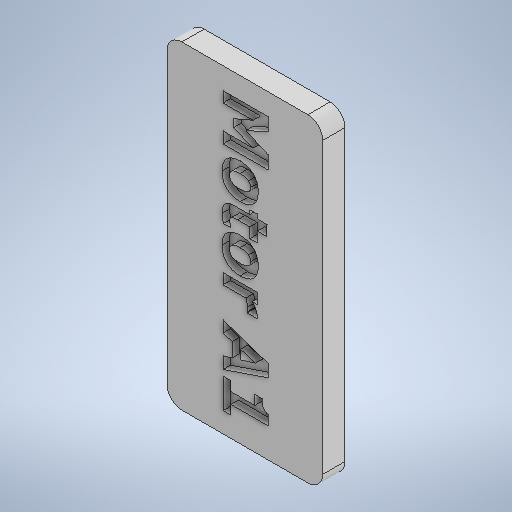
# Autodesk Inventor part: tag_lm2596_lid
Saved by Autodesk Inventor 2025 (Build 290162000, 162)
## iProperties
Created: 2025-01-26
Part Number: tag_lm2596_lid
Material: Všeobecné
Document SubType Name: Modeling
Designer: lukas
Density: 1 g/cm^3
Appearance: Výchozí
Author: lukas
Autodesk Inventor part; units mm, degrees
ref_plane "YZ Plane" through (0, 0, 0) normal (1, 0, 0) x (0, 1, 0)
ref_plane "XZ Plane" through (0, 0, 0) normal (0, 1, 0) x (-1, 0, 0)
ref_plane "XY Plane" through (0, 0, 0) normal (0, 0, 1) x (1, 0, 0)
sketch "Náčrt1" plane through (0, 0, 0) normal (0, 0, 1) x (1, 0, 0)
  line L0 (0, 30.1) -> (0, -30.1) projected
  line L1 (-14.7, 0) -> (14.7, 0) projected
  line L2 (-10.5, 21.5) -> (10.5, 21.5)
  line L3 (10.5, 21.5) -> (10.5, -21.5)
  line L4 (10.5, -21.5) -> (-10.5, -21.5)
  line L5 (-10.5, -21.5) -> (-10.5, 21.5)
  point P0 (0, 0)
  dimension "d0" = 21
  dimension "d1" = 43
  constraints: 8 end point, 2 parallel, 1 horizontal, 1 perpendicular, 2 other
  measures "d0" distance of L2.start L2.end
  measures "d1" distance of L2.end L3.end
extrude "Vysunutí1" add sketch "Náčrt1" along normal blind 3
sketch "Náčrt2" plane through (0, 0, 3) normal (0, 0, 1) x (1, 0, 0)
  line L0 (-10.5, -21.5) -> (10.5, -21.5) projected
  line L1 (10.5, -21.5) -> (10.5, 21.5) projected
  line L2 (10.5, 21.5) -> (-10.5, 21.5) projected
  line L3 (-10.5, 21.5) -> (-10.5, -21.5) projected
  line L4 (0, 30.1123) -> (0, -30.1736) projected
  line L5 (-14.7, 0) -> (14.7, 0) projected
  line L6 (7.4769, 21.5) -> (7.4769, -21.5614) construction
  line L7 (7.4769, -21.5614) -> (-7.39, -21.5614) construction
  line L8 (-7.39, -21.5614) -> (-7.39, 21.5) construction
  line L9 (-7.39, 21.5) -> (7.4769, 21.5) construction
  line L10 (-2.9423, 12.3646) -> (-2.9423, 13.8871)
  line L11 (-2.9423, 13.8871) -> (1.1013, 13.8871)
  line L12 (1.1013, 13.8871) -> (-1.5087, 14.9944)
  line L13 (-1.5087, 14.9944) -> (-1.5087, 16.0424)
  line L14 (-1.5087, 16.0424) -> (1.1013, 17.1497)
  line L15 (1.1013, 17.1497) -> (-2.9423, 17.1497)
  line L16 (-2.9423, 17.1497) -> (-2.9423, 18.5931)
  line L17 (-2.9423, 18.5931) -> (3.1577, 18.5931)
  line L18 (3.1577, 18.5931) -> (3.1577, 16.8284)
  line L19 (3.1577, 16.8284) -> (0.1473, 15.4739)
  line L20 (0.1473, 15.4739) -> (3.1577, 14.1293)
  line L21 (3.1577, 14.1293) -> (3.1577, 12.3646)
  line L22 (3.1577, 12.3646) -> (-2.9423, 12.3646)
  spline S0 degree 2 poles (-0.6436, 6.7688) (-1.7806, 6.7688) (-3.0856, 8.0096) (-3.0856, 9.1416) knots 0 0 0 1 2 2 2
  spline S1 degree 2 poles (-3.0856, 9.1416) (-3.0856, 10.2686) (-1.7806, 11.5193) (-0.6436, 11.5193) knots 0 0 0 1 2 2 2
  spline S2 degree 2 poles (-0.6436, 11.5193) (0.5032, 11.5193) (1.8033, 10.2686) (1.8033, 9.1416) knots 0 0 0 1 2 2 2
  spline S3 degree 2 poles (1.8033, 9.1416) (1.8033, 8.0145) (0.4983, 6.7688) (-0.6436, 6.7688) knots 0 0 0 1 2 2 2
  spline S4 degree 2 poles (-0.6535, 8.2369) (-0.2432, 8.2369) (0.3055, 8.3704) (0.4686, 8.489) knots 0 0 0 1 2 2 2
  spline S5 degree 2 poles (0.4686, 8.489) (0.6416, 8.6176) (0.7751, 8.9389) (0.7751, 9.1416) knots 0 0 0 1 2 2 2
  spline S6 degree 2 poles (0.7751, 9.1416) (0.7751, 9.3393) (0.6564, 9.6507) (0.4884, 9.7792) knots 0 0 0 1 2 2 2
  spline S7 degree 2 poles (0.4884, 9.7792) (0.3302, 9.9028) (-0.2284, 10.0511) (-0.6535, 10.0511) knots 0 0 0 1 2 2 2
  spline S8 degree 2 poles (-0.6535, 10.0511) (-1.0737, 10.0511) (-1.5928, 9.9127) (-1.7509, 9.799) knots 0 0 0 1 2 2 2
  spline S9 degree 2 poles (-1.7509, 9.799) (-1.9091, 9.6853) (-2.0574, 9.3393) (-2.0574, 9.1317) knots 0 0 0 1 2 2 2
  spline S10 degree 2 poles (-2.0574, 9.1317) (-2.0574, 8.9587) (-1.9091, 8.6027) (-1.7608, 8.494) knots 0 0 0 1 2 2 2
  spline S11 degree 2 poles (-1.7608, 8.494) (-1.5878, 8.3704) (-1.0885, 8.2369) (-0.6535, 8.2369) knots 0 0 0 1 2 2 2
  spline S12 degree 2 poles (-3.0312, 4.2477) (-3.0312, 5.1227) (-2.3095, 5.9235) (-1.4889, 5.9235) knots 0 0 0 1 2 2 2
  line L23 (-1.4889, 5.9235) -> (0.6614, 5.9235)
  line L24 (0.6614, 5.9235) -> (0.6614, 6.4722)
  line L25 (0.6614, 6.4722) -> (1.6599, 6.4722)
  line L26 (1.6599, 6.4722) -> (1.6599, 5.9235)
  line L27 (1.6599, 5.9235) -> (2.9748, 5.9235)
  line L28 (2.9748, 5.9235) -> (2.9748, 4.4899)
  line L29 (2.9748, 4.4899) -> (1.6599, 4.4899)
  line L30 (1.6599, 4.4899) -> (1.6599, 3.1058)
  line L31 (1.6599, 3.1058) -> (0.6614, 3.1058)
  line L32 (0.6614, 3.1058) -> (0.6614, 4.4899)
  line L33 (0.6614, 4.4899) -> (-0.9748, 4.4899)
  spline S13 degree 2 poles (-0.9748, 4.4899) (-1.2171, 4.4899) (-1.5779, 4.4801) (-1.7213, 4.4207) knots 0 0 0 1 2 2 2
  spline S14 degree 2 poles (-1.7213, 4.4207) (-1.8646, 4.3614) (-2.0327, 4.0698) (-2.0327, 3.7929) knots 0 0 0 1 2 2 2
  spline S15 degree 2 poles (-2.0327, 3.7929) (-2.0327, 3.6743) (-1.9338, 3.3036) (-1.8943, 3.2294) knots 0 0 0 1 2 2 2
  line L34 (-1.8943, 3.2294) -> (-1.8943, 3.1058)
  line L35 (-1.8943, 3.1058) -> (-2.9027, 3.1058)
  spline S16 degree 2 poles (-2.9027, 3.1058) (-2.962, 3.3382) (-3.0312, 3.8621) (-3.0312, 4.2477) knots 0 0 0 1 2 2 2
  spline S17 degree 2 poles (-0.6436, -1.8918) (-1.7806, -1.8918) (-3.0856, -0.6511) (-3.0856, 0.4809) knots 0 0 0 1 2 2 2
  spline S18 degree 2 poles (-3.0856, 0.4809) (-3.0856, 1.608) (-1.7806, 2.8587) (-0.6436, 2.8587) knots 0 0 0 1 2 2 2
  spline S19 degree 2 poles (-0.6436, 2.8587) (0.5032, 2.8587) (1.8033, 1.608) (1.8033, 0.4809) knots 0 0 0 1 2 2 2
  spline S20 degree 2 poles (1.8033, 0.4809) (1.8033, -0.6461) (0.4983, -1.8918) (-0.6436, -1.8918) knots 0 0 0 1 2 2 2
  spline S21 degree 2 poles (-0.6535, -0.4237) (-0.2432, -0.4237) (0.3055, -0.2902) (0.4686, -0.1716) knots 0 0 0 1 2 2 2
  spline S22 degree 2 poles (0.4686, -0.1716) (0.6416, -0.043) (0.7751, 0.2783) (0.7751, 0.4809) knots 0 0 0 1 2 2 2
  spline S23 degree 2 poles (0.7751, 0.4809) (0.7751, 0.6787) (0.6564, 0.9901) (0.4884, 1.1186) knots 0 0 0 1 2 2 2
  spline S24 degree 2 poles (0.4884, 1.1186) (0.3302, 1.2422) (-0.2284, 1.3905) (-0.6535, 1.3905) knots 0 0 0 1 2 2 2
  spline S25 degree 2 poles (-0.6535, 1.3905) (-1.0737, 1.3905) (-1.5928, 1.2521) (-1.7509, 1.1384) knots 0 0 0 1 2 2 2
  spline S26 degree 2 poles (-1.7509, 1.1384) (-1.9091, 1.0247) (-2.0574, 0.6787) (-2.0574, 0.4711) knots 0 0 0 1 2 2 2
  spline S27 degree 2 poles (-2.0574, 0.4711) (-2.0574, 0.298) (-1.9091, -0.0579) (-1.7608, -0.1666) knots 0 0 0 1 2 2 2
  spline S28 degree 2 poles (-1.7608, -0.1666) (-1.5878, -0.2902) (-1.0885, -0.4237) (-0.6535, -0.4237) knots 0 0 0 1 2 2 2
  line L36 (0.3005, -5.7426) -> (0.3005, -5.624)
  spline S29 degree 2 poles (0.3005, -5.624) (0.3302, -5.54) (0.3598, -5.2285) (0.3598, -5.0407) knots 0 0 0 1 2 2 2
  spline S30 degree 2 poles (0.3598, -5.0407) (0.3598, -4.8182) (0.2264, -4.319) (0.1374, -4.0866) knots 0 0 0 1 2 2 2
  line L37 (0.1374, -4.0866) -> (-2.9423, -4.0866)
  line L38 (-2.9423, -4.0866) -> (-2.9423, -2.6531)
  line L39 (-2.9423, -2.6531) -> (1.6599, -2.6531)
  line L40 (1.6599, -2.6531) -> (1.6599, -4.0866)
  line L41 (1.6599, -4.0866) -> (0.9975, -4.0866)
  spline S31 degree 2 poles (0.9975, -4.0866) (1.0865, -4.1855) (1.3633, -4.5315) (1.4474, -4.6749) knots 0 0 0 1 2 2 2
  spline S32 degree 2 poles (1.4474, -4.6749) (1.5413, -4.8331) (1.6748, -5.2483) (1.6748, -5.4312) knots 0 0 0 1 2 2 2
  spline S33 degree 2 poles (1.6748, -5.4312) (1.6748, -5.5004) (1.6649, -5.6734) (1.6599, -5.7426) knots 0 0 0 1 2 2 2
  line L42 (1.6599, -5.7426) -> (0.3005, -5.7426)
  line L43 (-2.9423, -8.1747) -> (3.1577, -10.2361)
  line L44 (3.1577, -10.2361) -> (3.1577, -11.9069)
  line L45 (3.1577, -11.9069) -> (-2.9423, -13.9682)
  line L46 (-2.9423, -13.9682) -> (-2.9423, -12.3913)
  line L47 (-2.9423, -12.3913) -> (-1.6966, -12.0107)
  line L48 (-1.6966, -12.0107) -> (-1.6966, -10.0927)
  line L49 (-1.6966, -10.0927) -> (-2.9423, -9.7071)
  line L50 (-2.9423, -9.7071) -> (-2.9423, -8.1747)
  line L51 (-0.5893, -11.6746) -> (1.4276, -11.0517)
  line L52 (1.4276, -11.0517) -> (-0.5893, -10.4239)
  line L53 (-0.5893, -10.4239) -> (-0.5893, -11.6746)
  line L54 (-2.9423, -18.7731) -> (-2.9423, -14.7443)
  line L55 (-2.9423, -14.7443) -> (-1.8795, -14.7443)
  line L56 (-1.8795, -14.7443) -> (-1.8795, -16.0296)
  line L57 (-1.8795, -16.0296) -> (1.3485, -16.0296)
  line L58 (1.3485, -16.0296) -> (1.3485, -14.7443)
  line L59 (1.3485, -14.7443) -> (2.3421, -14.7443)
  spline S34 degree 2 poles (2.3421, -14.7443) (2.3421, -15.0261) (2.4162, -15.5847) (2.4953, -15.7528) knots 0 0 0 1 2 2 2
  spline S35 degree 2 poles (2.4953, -15.7528) (2.5942, -15.9456) (2.9254, -16.1631) (3.1726, -16.1828) knots 0 0 0 1 2 2 2
  line L60 (3.1726, -16.1828) -> (3.1726, -17.5175)
  line L61 (3.1726, -17.5175) -> (-1.8795, -17.5175)
  line L62 (-1.8795, -17.5175) -> (-1.8795, -18.7731)
  line L63 (-1.8795, -18.7731) -> (-2.9423, -18.7731)
  point P0 (0, 0)
  constraints: 1 point on line, 2 other
extrude "Vysunutí2" cut sketch "Náčrt2" against normal blind 1 contours L61 L62 L63 L54 L55 L56 L57 L4 | L4 L57 L58 L59 S34 S35 L60 L61 | S17 S18 S19 L4 S24 S25 S26 S27 L5 | L5 S27 S28 S21 L4 S20 S17 | S20 L4 S21 S22 L5 | L5 S22 S23 S24 L4 S19 S20 | L45 L46 L47 L48 L49 L50 L43 L4 L52 L53 L51 | L4 L51 L52 L43 L44 L45 | L17 L18 L19 L20 L21 L22 L4 L11 L12 L14 L15 | L4 L15 L16 L17 | L39 L40 L41 S31 S32 S33 L42 L36 S29 S30 L37 L4 | L4 L37 L38 L39 | L4 L12 L13 L14 | L33 S13 S14 S15 L34 L35 S16 S12 L23 L4 | L4 L23 L24 L25 L26 L27 L28 L29 L30 L31 L32 L33 | L4 L22 L10 L11 | S3 S0 S1 S2 L4 S7 S8 S9 S10 S11 S4 | L4 S4 S5 S6 S7 S2 S3
fillet "Zaoblení1" radius 2 4 edges at (-10.5, -21.5, 1.5) (10.5, -21.5, 1.5) (10.5, 21.5, 1.5) (-10.5, 21.5, 1.5)
